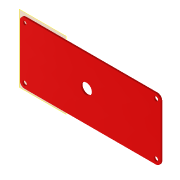
# Autodesk Inventor part: ESP32ParasiteMicroscope_top_v0
Saved by Autodesk Inventor 2022 (Build 260153000, 153)
## iProperties
Created: 2022-02-02
Part Number: ESP32ParasiteMicroscope_top_v0
Material: Generisch
Document SubType Name: Modeling
Designer: diederichbenedict
Density: 1 g/cm^3
Appearance: Rot
Author: diederichbenedict
Autodesk Inventor part; units mm, degrees
ref_plane "YZ Plane" through (0, 0, 0) normal (1, 0, 0) x (0, 1, 0)
ref_plane "XZ Plane" through (0, 0, 0) normal (0, 1, 0) x (-1, 0, 0)
ref_plane "XY Plane" through (0, 0, 0) normal (0, 0, 1) x (1, 0, 0)
ref_plane "Arbeitsebene1" through (0, 0, 0) normal (0, 0, 1) x (1, 0, 0)
sketch "Skizze1" plane through (0, 0, 0) normal (0, 0, 1) x (1, 0, 0)
  line L0 (-37.75, 12.7) -> (-37.75, -12.7)
  spline S0 degree 3 poles (-24.9439, 0) (-24.9647, 2.9337) (-24.4115, 5.8432) (-22.6462, 10.2329) (-21.7787, 11.8145) (-19.8669, 14.4875) (-18.8837, 15.6093) (-17.7982, 16.626) knots 0 0 0 0 0.880121 0.880121 1.419326 1.419326 1.865938 1.865938 1.865938 1.865938
  arc A0 (-17.7982, 16.626) -> (-19.6031, 19.4874) centre (-19.6031, 17.4874) ccw
  line L1 (-19.6031, 19.4874) -> (-41.5374, 19.4874)
  arc A1 (-41.5374, 19.4874) -> (-44.5374, 16.4874) centre (-41.5374, 16.4874) ccw
  line L2 (-44.5374, 16.4874) -> (-44.5374, -16.4874)
  arc A2 (-44.5374, -16.4874) -> (-41.5374, -19.4874) centre (-41.5374, -16.4874) ccw
  line L3 (-41.5374, -19.4874) -> (-19.6031, -19.4874)
  arc A3 (-19.6031, -19.4874) -> (-17.7982, -16.626) centre (-19.6031, -17.4874) ccw
  spline S1 degree 3 poles (-17.7982, -16.626) (-19.7157, -14.83) (-21.3076, -12.712) (-23.3127, -8.7647) (-23.9319, -7.0725) (-24.755, -3.5801) (-24.9566, -1.7925) (-24.9439, 0) knots 0.093538 0.093538 0.093538 0.093538 0.883139 0.883139 1.421841 1.421841 1.959644 1.959644 1.959644 1.959644
  circle A4 centre (-41.5374, 16.4874) radius 1.15
  circle A5 centre (-41.5374, -16.4874) radius 1.4
  spline S2 degree 3 poles (16.0826, -13.4603) (15.1069, -14.7838) (13.9918, -15.9978) (12.757, -17.0814) knots 0 0 0 0 1 1 1 1
  arc A6 (12.757, -17.0814) -> (14.7153, -19.4874) centre (14.7153, -17.4874) ccw
  line L4 (14.7153, -19.4874) -> (41.5374, -19.4874)
  arc A7 (41.5374, -19.4874) -> (44.5374, -16.4874) centre (41.5374, -16.4874) ccw
  line L5 (44.5374, -16.4874) -> (44.5374, 16.4874)
  arc A8 (44.5374, 16.4874) -> (41.5374, 19.4874) centre (41.5374, 16.4874) ccw
  line L6 (41.5374, 19.4874) -> (14.7153, 19.4874)
  arc A9 (14.7153, 19.4874) -> (12.757, 17.0814) centre (14.7153, 17.4874) ccw
  spline S3 degree 3 poles (12.757, 17.0814) (13.9918, 15.9978) (15.1069, 14.7838) (16.0826, 13.4603) knots 0 0 0 0 1 1 1 1
  arc A10 (16.0826, -13.4603) -> (16.0826, 13.4603) centre (-2.4439, 0) ccw
  circle A11 centre (41.5374, 16.4874) radius 1.4
  circle A12 centre (41.5374, -16.4874) radius 1.4
  line L7 (-19.6031, 19.4874) -> (14.7153, 19.4874)
  line L8 (14.7153, -19.4874) -> (-19.6031, -19.4874)
  circle A13 centre (-2.4439, 0) radius 3.45
  point P0 (0, 0)
  constraints: 4 end point, 1 horizontal, 1 parallel, 1 tangent
extrude "Extrusion1" add sketch "Skizze1" along normal blind 1
